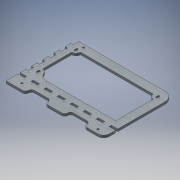
# Autodesk Inventor part: LatoAlimentatore
Saved by Autodesk Inventor 2018.3 (Build 223284000, 284)
## iProperties
Created: 2019-03-05
Part Number: LatoAlimentatore
Material: Generico
Document SubType Name: Modeling
Designer: AlfyPc
Density: 1 g/cm^3
Appearance: Legno - Verniciato - Bianco
Author: AlfyPc
Autodesk Inventor part; units mm, degrees
ref_plane "YZ Plane" through (0, 0, 0) normal (1, 0, 0) x (0, 1, 0)
ref_plane "XZ Plane" through (0, 0, 0) normal (0, 1, 0) x (-1, 0, 0)
ref_plane "XY Plane" through (0, 0, 0) normal (0, 0, 1) x (1, 0, 0)
sketch "Schizzo1" plane through (0, 0, 0) normal (0, 0, 1) x (1, 0, 0)
  line L0 (-152.5, 86) -> (-2.5, 86) construction
  line L1 (-152.5, 0) -> (-152.5, 86) construction
  line L2 (-2.5, 0) -> (-2.5, 86) construction
  circle A0 centre (-9.5, 81) radius 1.5 projected
  circle A1 centre (-147.5, 81) radius 1.5 projected
  circle A2 centre (-147.5, 17) radius 1.5 projected
  line L3 (4, 95) -> (-161, 95)
  line L4 (-161, -24) -> (-133, -24)
  line L5 (-128, -19) -> (-128, -19)
  line L6 (-123, -14) -> (-100, -14)
  line L7 (-95, -19) -> (-95, -19)
  line L8 (-90, -24) -> (-67, -24)
  line L9 (-62, -19) -> (-62, -19)
  line L10 (-57, -14) -> (-34, -14)
  line L11 (-29, -19) -> (-29, -19)
  line L12 (-24, -24) -> (4, -24)
  arc A3 (-133, -24) -> (-128, -19) centre (-133, -19) ccw
  arc A4 (-123, -14) -> (-128, -19) centre (-123, -19) ccw
  arc A5 (-95, -19) -> (-100, -14) centre (-100, -19) ccw
  arc A6 (-95, -19) -> (-90, -24) centre (-90, -19) ccw
  arc A7 (-67, -24) -> (-62, -19) centre (-67, -19) ccw
  arc A8 (-57, -14) -> (-62, -19) centre (-57, -19) ccw
  arc A9 (-29, -19) -> (-34, -14) centre (-34, -19) ccw
  arc A10 (-29, -19) -> (-24, -24) centre (-24, -19) ccw
  arc A11 (-17, 81) -> (-9.5, 73.5) centre (-9.5, 81) ccw
  arc A12 (-147.5, 73.5) -> (-140, 81) centre (-147.5, 81) ccw
  arc A13 (-140.4901, 19.6667) -> (-147.5, 24.5) centre (-147.5, 17) ccw
  line L13 (-147.5, 73.5) -> (-147.5, 24.5)
  line L14 (-17, 81) -> (-140, 81)
  line L15 (-9.5, 10) -> (-126.4703, 10)
  arc A14 (-140.4901, 19.6667) -> (-126.4703, 10) centre (-126.4703, 25) ccw
  line L16 (-9.5, 10) -> (-9.5, 73.5)
  line L17 (-161, 95) -> (-161, -24)
  line L18 (4, 95) -> (4, -24)
  line L19 (-161, -4) -> (-150, -4) projected
  line L20 (-150, 0) -> (-150, -4) projected
  line L21 (-150, 0) -> (-161, 0) projected
  line L22 (-161, 0) -> (-161, -4) projected
  line L23 (-139, -4) -> (-128, -4) projected
  line L24 (-128, 0) -> (-128, -4) projected
  line L25 (-128, 0) -> (-139, 0) projected
  line L26 (-139, 0) -> (-139, -4) projected
  line L27 (-117, -4) -> (-106, -4) projected
  line L28 (-106, 0) -> (-106, -4) projected
  line L29 (-106, 0) -> (-117, 0) projected
  line L30 (-117, 0) -> (-117, -4) projected
  line L31 (-95, -4) -> (-84, -4) projected
  line L32 (-84, 0) -> (-84, -4) projected
  line L33 (-84, 0) -> (-95, 0) projected
  line L34 (-95, 0) -> (-95, -4) projected
  line L35 (-73, -4) -> (-62, -4) projected
  line L36 (-62, 0) -> (-62, -4) projected
  line L37 (-62, 0) -> (-73, 0) projected
  line L38 (-73, 0) -> (-73, -4) projected
  line L39 (-51, -4) -> (-40, -4) projected
  line L40 (-40, 0) -> (-40, -4) projected
  line L41 (-40, 0) -> (-51, 0) projected
  line L42 (-51, 0) -> (-51, -4) projected
  line L43 (-29, -4) -> (-18, -4) projected
  line L44 (-18, 0) -> (-18, -4) projected
  line L45 (-18, 0) -> (-29, 0) projected
  line L46 (-29, 0) -> (-29, -4) projected
  line L47 (-7, -4) -> (4, -4) projected
  line L48 (-7, 0) -> (-7, -4) projected
  line L49 (-147.5, 82.5) -> (-147.5, 79.5) construction
  line L50 (-149, 82.5) -> (-149, 79.5)
  line L51 (-146, 79.5) -> (-146, 82.5)
  arc A15 (-146, 82.5) -> (-149, 82.5) centre (-147.5, 82.5) ccw
  arc A16 (-149, 79.5) -> (-146, 79.5) centre (-147.5, 79.5) ccw
  line L52 (-9.5, 82.5) -> (-9.5, 79.5) construction
  line L53 (-11, 82.5) -> (-11, 79.5)
  line L54 (-8, 79.5) -> (-8, 82.5)
  arc A17 (-8, 82.5) -> (-11, 82.5) centre (-9.5, 82.5) ccw
  arc A18 (-11, 79.5) -> (-8, 79.5) centre (-9.5, 79.5) ccw
  line L55 (-147.5, 18.5) -> (-147.5, 15.5) construction
  line L56 (-149, 18.5) -> (-149, 15.5)
  line L57 (-146, 15.5) -> (-146, 18.5)
  arc A19 (-146, 18.5) -> (-149, 18.5) centre (-147.5, 18.5) ccw
  arc A20 (-149, 15.5) -> (-146, 15.5) centre (-147.5, 15.5) ccw
  line L58 (4, 0) -> (4, -4) projected
  line L59 (4, 0) -> (-7, 0) projected
  point P0 (-128, -24)
  point P1 (-128, -14)
  point P2 (-95, -14)
  point P3 (-95, -24)
  point P4 (-62, -24)
  point P5 (-62, -14)
  point P6 (-29, -14)
  point P7 (-29, -24)
  point P8 (-144.8074, 10)
  dimension "d0" = 165
  dimension "d9" = 33
  dimension "d10" = 10
  dimension "d11" = 33
  dimension "d12" = 10
  dimension "d13" = 33
  dimension "d14" = 10
  dimension "d15" = 33
  dimension "d16" = 5
  dimension "d21" = 15
  constraints: 62 end point, 43 point on circle, 30 tangent, 21 point on line, 18 centre point, 7 equal radius, 7 perpendicular, 4 parallel, 3 horizontal, 3 midpoint, 2 coincident, 2 vertical
  measures "d0" distance of L3.end L3.start
  measures "d9" distance of L4.start point (-128, -24)
  measures "d10" distance of point (-128, -24) point (-128, -14)
  measures "d11" distance of point (-128, -14) point (-95, -14)
  measures "d12" distance of point (-95, -14) point (-95, -24)
  measures "d13" distance of point (-95, -24) point (-62, -24)
  measures "d14" distance of point (-62, -24) point (-62, -14)
  measures "d15" distance of point (-62, -14) point (-29, -14)
  measures "d16" radius of A3
  measures "d21" radius of A14
extrude "Estrusione1" add sketch "Schizzo1" along normal blind 4 contours L18 L59 L48 L47 L12 A10 A9 L10 A8 A7 L8 A6 A5 L6 A4 A3 L4 L17 L19 L20 L21 L3
sketch "Schizzo2" plane through (0, 0, 4) normal (0, 0, 1) x (1, 0, 0)
  line L0 (-157, 85.5) -> (-161, 85.5)
  line L1 (-161, 85.5) -> (-161, 95)
  line L2 (-161, 95) -> (-157, 95)
  line L3 (-157, 95) -> (-157, 85.5)
  line L4 (-157, 66.5) -> (-161, 66.5)
  line L5 (-161, 66.5) -> (-161, 76)
  line L6 (-161, 76) -> (-157, 76)
  line L7 (-157, 76) -> (-157, 66.5)
  line L8 (-161, 57) -> (-157, 57)
  line L9 (-157, 57) -> (-157, 47.5)
  line L10 (-157, 47.5) -> (-161, 47.5)
  line L11 (-161, 47.5) -> (-161, 57)
  line L12 (-157, 28.5) -> (-161, 28.5)
  line L13 (-161, 28.5) -> (-161, 38)
  line L14 (-161, 38) -> (-157, 38)
  line L15 (-157, 38) -> (-157, 28.5)
  line L16 (-161, 19) -> (-157, 19)
  line L17 (-157, 19) -> (-157, 9.5)
  line L18 (-157, 9.5) -> (-161, 9.5)
  line L19 (-161, 9.5) -> (-161, 19)
  point P0 (0, 0)
  constraints: 40 end point, 10 horizontal, 10 vertical, 20 other
extrude "Estrusione2" cut sketch "Schizzo2" against normal blind 4
fillet "Raccordo1" radius 15 1 edges at (4, 95, 2)
fillet "Raccordo2" radius 10 1 edges at (4, -24, 2)
sketch "Schizzo3" plane through (0, 0, 4) normal (0, 0, 1) x (1, 0, 0)
  line L0 (-14.15, 0) -> (-10.85, 0) projected
  line L1 (-146.15, 0) -> (-142.85, 0) projected
  line L2 (-144.5, 0) -> (-137.5, 0) construction
  line L3 (-12.5, 0) -> (-12.5, -17) construction
  circle A0 centre (-12.5, -17) radius 1.65
  line L4 (-157, 82.4) -> (-157, 79.1) construction
  line L5 (-157, 85.5) -> (-157, 95) construction
  line L6 (-157, 95) -> (-157, 85.5) projected
  line L7 (-157, 90.25) -> (-144, 90.25) construction
  circle A1 centre (-144, 90.25) radius 1.65
  line L8 (-157, -12.35) -> (-157, -15.65) construction
  line L9 (-157, -14) -> (-144, -14) construction
  circle A2 centre (-144, -14) radius 1.65
  point P0 (0, 0)
  dimension "d32" = 3.3
  dimension "d35" = 13
  dimension "d36" = 3.3
  dimension "d37" = 13
  dimension "d38" = 3.3
  dimension "d39" = 17
  constraints: 8 end point, 4 midpoint, 3 centre point, 3 coincident, 3 horizontal, 1 vertical
  measures "d32" diameter of A0
  measures "d35" distance of L7.start L7.end
  measures "d36" diameter of A1
  measures "d37" distance of L9.start L9.end
  measures "d38" diameter of A2
  measures "d39" distance of L3.start L3.end
extrude "Estrusione3" cut sketch "Schizzo3" against normal blind 4
